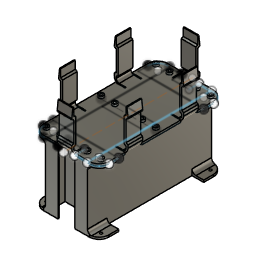
wall_holder (Autodesk Fusion 360 design; units mm, degrees)
Autodesk Fusion 360 part; units mm, degrees
other "Grundnetzelement1"
sketch "Skizze2" plane through (0, 0, 0) normal (0, 0, 1) x (1, 0, 0)
  line L0 (67, -14.1187) -> (67, 146.9687) construction
  line L1 (124.2467, 81.5) -> (-73.8076, 81.5) construction
  line L2 (90.5, 18) -> (43.5, 18)
  line L3 (33.5, 28) -> (33.5, 135)
  line L4 (43.5, 145) -> (90.5, 145)
  line L5 (100.5, 135) -> (100.5, 28)
  line L6 (31.5, 102.5) -> (35.5, 102.5)
  line L7 (35.5, 102.5) -> (35.5, 117.5)
  line L8 (35.5, 117.5) -> (31.5, 117.5)
  line L9 (31.5, 117.5) -> (31.5, 102.5)
  line L10 (59.5, 20) -> (74.5, 20)
  line L11 (74.5, 20) -> (74.5, 16)
  line L12 (74.5, 16) -> (59.5, 16)
  line L13 (59.5, 16) -> (59.5, 20)
  line L14 (35.5, 45.5) -> (31.5, 45.5)
  line L15 (31.5, 45.5) -> (31.5, 60.5)
  line L16 (35.5, 60.5) -> (35.5, 45.5)
  line L17 (31.5, 60.5) -> (35.5, 60.5)
  line L18 (59.5, 147) -> (59.5, 143)
  line L19 (59.5, 143) -> (74.5, 143)
  line L20 (74.5, 143) -> (74.5, 147)
  line L21 (74.5, 147) -> (59.5, 147)
  line L22 (98.5, 102.5) -> (98.5, 117.5)
  line L23 (102.5, 117.5) -> (102.5, 102.5)
  line L24 (98.5, 117.5) -> (102.5, 117.5)
  line L25 (102.5, 102.5) -> (98.5, 102.5)
  line L26 (102.5, 60.5) -> (98.5, 60.5)
  line L27 (98.5, 60.5) -> (98.5, 45.5)
  line L28 (102.5, 45.5) -> (102.5, 60.5)
  line L29 (98.5, 45.5) -> (102.5, 45.5)
  arc A0 (43.5, 145) -> (33.5, 135) centre (43.5, 135) ccw
  arc A1 (100.5, 135) -> (90.5, 145) centre (90.5, 135) ccw
  arc A2 (90.5, 18) -> (100.5, 28) centre (90.5, 28) ccw
  arc A3 (33.5, 28) -> (43.5, 18) centre (43.5, 28) ccw
  circle A4 centre (39, 137.5) radius 2.5
  circle A5 centre (39, 137.5) radius 4.5
  circle A6 centre (53, 137.5) radius 2.5
  circle A7 centre (53, 137.5) radius 4.5
  circle A8 centre (39, 109.5) radius 2.5
  circle A9 centre (39, 109.5) radius 4.5
  circle A10 centre (53, 109.5) radius 2.5
  circle A11 centre (53, 109.5) radius 4.5
  circle A12 centre (39, 81.5) radius 2.5
  circle A13 centre (39, 81.5) radius 4.5
  circle A14 centre (53, 81.5) radius 2.5
  circle A15 centre (53, 81.5) radius 4.5
  circle A16 centre (39, 53.5) radius 2.5
  circle A17 centre (39, 53.5) radius 4.5
  circle A18 centre (53, 53.5) radius 2.5
  circle A19 centre (53, 53.5) radius 4.5
  circle A20 centre (39, 25.5) radius 2.5
  circle A21 centre (39, 25.5) radius 4.5
  circle A22 centre (53, 25.5) radius 2.5
  circle A23 centre (53, 25.5) radius 4.5
  line L30 (41, 137.5) -> (37, 137.5)
  line L31 (37, 137.5) -> (37, 25.5)
  line L32 (37, 25.5) -> (41, 25.5)
  line L33 (41, 25.5) -> (41, 137.5)
  line L34 (39, 137.5) -> (39, 109.5) construction
  line L35 (59.5, 145) -> (58.5, 145)
  line L36 (58.5, 145) -> (58.5, 135)
  line L37 (58.5, 135) -> (59.5, 135)
  line L38 (59.5, 135) -> (59.5, 145)
  line L39 (74.5, 145) -> (75.5, 145)
  line L40 (75.5, 145) -> (75.5, 135)
  line L41 (75.5, 135) -> (74.5, 135)
  line L42 (74.5, 135) -> (74.5, 145)
  line L43 (74.5, 28) -> (74.5, 18)
  line L44 (75.5, 18) -> (75.5, 28)
  line L45 (58.5, 18) -> (58.5, 28)
  line L46 (59.5, 28) -> (59.5, 18)
  line L47 (58.5, 28) -> (59.5, 28)
  line L48 (59.5, 18) -> (58.5, 18)
  line L49 (74.5, 18) -> (75.5, 18)
  line L50 (75.5, 28) -> (74.5, 28)
  line L51 (33.5, 117.5) -> (43.5, 117.5)
  line L52 (43.5, 117.5) -> (43.5, 118.5)
  line L53 (43.5, 118.5) -> (33.5, 118.5)
  line L54 (33.5, 118.5) -> (33.5, 117.5)
  line L55 (33.5, 102.5) -> (43.5, 102.5)
  line L56 (43.5, 102.5) -> (43.5, 101.5)
  line L57 (43.5, 101.5) -> (33.5, 101.5)
  line L58 (33.5, 101.5) -> (33.5, 102.5)
  line L59 (33.5, 61.5) -> (33.5, 60.5)
  line L60 (33.5, 60.5) -> (43.5, 60.5)
  line L61 (43.5, 61.5) -> (33.5, 61.5)
  line L62 (43.5, 60.5) -> (43.5, 61.5)
  line L63 (43.5, 45.5) -> (43.5, 44.5)
  line L64 (33.5, 45.5) -> (43.5, 45.5)
  line L65 (33.5, 44.5) -> (33.5, 45.5)
  line L66 (43.5, 44.5) -> (33.5, 44.5)
  line L67 (90.5, 101.5) -> (100.5, 101.5)
  line L68 (100.5, 102.5) -> (90.5, 102.5)
  line L69 (100.5, 101.5) -> (100.5, 102.5)
  line L70 (90.5, 102.5) -> (90.5, 101.5)
  line L71 (100.5, 118.5) -> (100.5, 117.5)
  line L72 (100.5, 117.5) -> (90.5, 117.5)
  line L73 (90.5, 118.5) -> (100.5, 118.5)
  line L74 (90.5, 117.5) -> (90.5, 118.5)
  line L75 (100.5, 60.5) -> (90.5, 60.5)
  line L76 (90.5, 61.5) -> (100.5, 61.5)
  line L77 (100.5, 61.5) -> (100.5, 60.5)
  line L78 (90.5, 60.5) -> (90.5, 61.5)
  line L79 (90.5, 44.5) -> (100.5, 44.5)
  line L80 (90.5, 45.5) -> (90.5, 44.5)
  line L81 (100.5, 45.5) -> (90.5, 45.5)
  line L82 (100.5, 44.5) -> (100.5, 45.5)
  circle A24 centre (67, 137.5) radius 2.5
  circle A25 centre (67, 137.5) radius 4.5
  circle A26 centre (81, 137.5) radius 2.5
  circle A27 centre (81, 137.5) radius 4.5
  circle A28 centre (95, 137.5) radius 2.5
  circle A29 centre (95, 137.5) radius 4.5
  circle A30 centre (67, 109.5) radius 2.5
  circle A31 centre (67, 109.5) radius 4.5
  circle A32 centre (81, 109.5) radius 2.5
  circle A33 centre (81, 109.5) radius 4.5
  circle A34 centre (95, 109.5) radius 2.5
  circle A35 centre (95, 109.5) radius 4.5
  circle A36 centre (67, 81.5) radius 2.5
  circle A37 centre (67, 81.5) radius 4.5
  circle A38 centre (81, 81.5) radius 2.5
  circle A39 centre (81, 81.5) radius 4.5
  circle A40 centre (95, 81.5) radius 2.5
  circle A41 centre (95, 81.5) radius 4.5
  circle A42 centre (67, 53.5) radius 2.5
  circle A43 centre (67, 53.5) radius 4.5
  circle A44 centre (81, 53.5) radius 2.5
  circle A45 centre (81, 53.5) radius 4.5
  circle A46 centre (95, 53.5) radius 2.5
  circle A47 centre (95, 53.5) radius 4.5
  circle A48 centre (67, 25.5) radius 2.5
  circle A49 centre (67, 25.5) radius 4.5
  circle A50 centre (81, 25.5) radius 2.5
  circle A51 centre (81, 25.5) radius 4.5
  circle A52 centre (95, 25.5) radius 2.5
  circle A53 centre (95, 25.5) radius 4.5
  line L83 (93, 137.5) -> (97, 137.5)
  line L84 (97, 137.5) -> (97, 25.5)
  line L85 (93, 25.5) -> (93, 137.5)
  line L86 (97, 25.5) -> (93, 25.5)
  line L87 (41, 134.5) -> (37, 134.5)
  line L88 (37, 134.5) -> (37, 140.5)
  line L89 (37, 140.5) -> (41, 140.5)
  line L90 (41, 140.5) -> (41, 134.5)
  line L91 (55, 134.5) -> (51, 134.5)
  line L92 (51, 134.5) -> (51, 140.5)
  line L93 (51, 140.5) -> (55, 140.5)
  line L94 (55, 140.5) -> (55, 134.5)
  line L95 (69, 134.5) -> (65, 134.5)
  line L96 (65, 134.5) -> (65, 140.5)
  line L97 (65, 140.5) -> (69, 140.5)
  line L98 (69, 140.5) -> (69, 134.5)
  line L99 (83, 134.5) -> (79, 134.5)
  line L100 (79, 134.5) -> (79, 140.5)
  line L101 (79, 140.5) -> (83, 140.5)
  line L102 (83, 140.5) -> (83, 134.5)
  line L103 (97, 134.5) -> (93, 134.5)
  line L104 (93, 134.5) -> (93, 140.5)
  line L105 (93, 140.5) -> (97, 140.5)
  line L106 (97, 140.5) -> (97, 134.5)
  line L107 (41, 106.5) -> (37, 106.5)
  line L108 (37, 106.5) -> (37, 112.5)
  line L109 (37, 112.5) -> (41, 112.5)
  line L110 (41, 112.5) -> (41, 106.5)
  line L111 (55, 106.5) -> (51, 106.5)
  line L112 (51, 106.5) -> (51, 112.5)
  line L113 (51, 112.5) -> (55, 112.5)
  line L114 (55, 112.5) -> (55, 106.5)
  line L115 (69, 106.5) -> (65, 106.5)
  line L116 (65, 106.5) -> (65, 112.5)
  line L117 (65, 112.5) -> (69, 112.5)
  line L118 (69, 112.5) -> (69, 106.5)
  line L119 (83, 106.5) -> (79, 106.5)
  line L120 (79, 106.5) -> (79, 112.5)
  line L121 (79, 112.5) -> (83, 112.5)
  line L122 (83, 112.5) -> (83, 106.5)
  line L123 (97, 106.5) -> (93, 106.5)
  line L124 (93, 106.5) -> (93, 112.5)
  line L125 (93, 112.5) -> (97, 112.5)
  line L126 (97, 112.5) -> (97, 106.5)
  line L127 (41, 78.5) -> (37, 78.5)
  line L128 (37, 78.5) -> (37, 84.5)
  line L129 (37, 84.5) -> (41, 84.5)
  line L130 (41, 84.5) -> (41, 78.5)
  line L131 (55, 78.5) -> (51, 78.5)
  line L132 (51, 78.5) -> (51, 84.5)
  line L133 (51, 84.5) -> (55, 84.5)
  line L134 (55, 84.5) -> (55, 78.5)
  line L135 (69, 78.5) -> (65, 78.5)
  line L136 (65, 78.5) -> (65, 84.5)
  line L137 (65, 84.5) -> (69, 84.5)
  line L138 (69, 84.5) -> (69, 78.5)
  line L139 (83, 78.5) -> (79, 78.5)
  line L140 (79, 78.5) -> (79, 84.5)
  line L141 (79, 84.5) -> (83, 84.5)
  line L142 (83, 84.5) -> (83, 78.5)
  line L143 (97, 78.5) -> (93, 78.5)
  line L144 (93, 78.5) -> (93, 84.5)
  line L145 (93, 84.5) -> (97, 84.5)
  line L146 (97, 84.5) -> (97, 78.5)
  line L147 (41, 50.5) -> (37, 50.5)
  line L148 (37, 50.5) -> (37, 56.5)
  line L149 (37, 56.5) -> (41, 56.5)
  line L150 (41, 56.5) -> (41, 50.5)
  line L151 (55, 50.5) -> (51, 50.5)
  line L152 (51, 50.5) -> (51, 56.5)
  line L153 (51, 56.5) -> (55, 56.5)
  line L154 (55, 56.5) -> (55, 50.5)
  line L155 (69, 50.5) -> (65, 50.5)
  line L156 (65, 50.5) -> (65, 56.5)
  line L157 (65, 56.5) -> (69, 56.5)
  line L158 (69, 56.5) -> (69, 50.5)
  line L159 (83, 50.5) -> (79, 50.5)
  line L160 (79, 50.5) -> (79, 56.5)
  line L161 (79, 56.5) -> (83, 56.5)
  line L162 (83, 56.5) -> (83, 50.5)
  line L163 (97, 50.5) -> (93, 50.5)
  line L164 (93, 50.5) -> (93, 56.5)
  line L165 (93, 56.5) -> (97, 56.5)
  line L166 (97, 56.5) -> (97, 50.5)
  line L167 (41, 22.5) -> (37, 22.5)
  line L168 (37, 22.5) -> (37, 28.5)
  line L169 (37, 28.5) -> (41, 28.5)
  line L170 (41, 28.5) -> (41, 22.5)
  line L171 (55, 22.5) -> (51, 22.5)
  line L172 (51, 22.5) -> (51, 28.5)
  line L173 (51, 28.5) -> (55, 28.5)
  line L174 (55, 28.5) -> (55, 22.5)
  line L175 (69, 22.5) -> (65, 22.5)
  line L176 (65, 22.5) -> (65, 28.5)
  line L177 (65, 28.5) -> (69, 28.5)
  line L178 (69, 28.5) -> (69, 22.5)
  line L179 (83, 22.5) -> (79, 22.5)
  line L180 (79, 22.5) -> (79, 28.5)
  line L181 (79, 28.5) -> (83, 28.5)
  line L182 (83, 28.5) -> (83, 22.5)
  line L183 (97, 22.5) -> (93, 22.5)
  line L184 (93, 22.5) -> (93, 28.5)
  line L185 (93, 28.5) -> (97, 28.5)
  line L186 (97, 28.5) -> (97, 22.5)
  point P0 (100.5, 18)
  point P1 (33.5, 18)
  point P2 (100.5, 145)
  point P3 (39, 137.5)
  point P4 (53, 137.5)
  point P5 (39, 109.5)
  point P6 (53, 109.5)
  point P7 (39, 81.5)
  point P8 (53, 81.5)
  point P9 (39, 53.5)
  point P10 (53, 53.5)
  point P11 (39, 25.5)
  point P12 (53, 25.5)
  point P13 (35.5, 60.5)
  point P14 (40.3584, 39.5)
  point P15 (35.5, 45.5)
  point P16 (98.5, 102.5)
  point P17 (93.6416, 123.5)
  point P18 (98.5, 117.5)
  point P19 (98.5, 60.5)
  point P20 (98.5, 60.5)
  point P21 (98.5, 45.5)
  point P22 (93.6416, 39.5)
  point P23 (102.5, 45.5)
  point P24 (98.5, 45.5)
  point P25 (93.6416, 36.5)
  point P26 (67, 137.5)
  point P27 (81, 137.5)
  point P28 (95, 137.5)
  point P29 (67, 109.5)
  point P30 (81, 109.5)
  point P31 (95, 109.5)
  point P32 (67, 81.5)
  point P33 (81, 81.5)
  point P34 (95, 81.5)
  point P35 (67, 53.5)
  point P36 (81, 53.5)
  point P37 (95, 53.5)
  point P38 (67, 25.5)
  point P39 (81, 25.5)
  point P40 (95, 25.5)
  dimension "d1" = 67
  dimension "d2" = 127
  dimension "d3" = 67
  dimension "d4" = 81.5
  dimension "d8" = 15
  dimension "d9" = 2
  dimension "d10" = 2
  dimension "d11" = 21
  dimension "d12" = 2
  dimension "d13" = 2
  dimension "d14" = 15
  dimension "d15" = 10
  dimension "d42" = 56
  dimension "d43" = -112
  dimension "d44" = 5
  dimension "d45" = 9
  dimension "d47" = 4
  dimension "d78" = 1
  dimension "d79" = 10
  dimension "d80" = 1
  dimension "d81" = 10
  dimension "d82" = 1
  dimension "d83" = 1
  dimension "d86" = 6
  constraint vertical L0
  constraint horizontal L1
  constraint horizontal L2
  constraint vertical L3
  constraint horizontal L4
  constraint vertical L5
  constraint symmetric L1 L2 L4
  constraint horizontal L6
  constraint vertical L7
  constraint horizontal L8
  constraint vertical L9
  constraint horizontal L10
  constraint vertical L11
  constraint horizontal L12
  constraint vertical L13
  constraint symmetric L1 L6.start L15.end
  constraint symmetric L1 L6.end P13
  constraint symmetric L1 L7.end P15
  constraint symmetric L1 L8.end L14.end
  constraint symmetric L1 L10.start L18.end
  constraint symmetric L1 L10.end L19.end
  constraint symmetric L1 L11.end L20.end
  constraint symmetric L1 L12.end L18.start
  constraint symmetric L0 L6.start L23.end
  constraint symmetric L0 L6.end P16
  constraint symmetric L0 L7.end P18
  constraint symmetric L0 L8.end L23.start
  constraint symmetric L0 P15 P24
  constraint symmetric L0 L14.end P23
  constraint symmetric L0 L15.end L26.start
  constraint symmetric L0 P13 P20
  constraint tangent L4 A0
  constraint tangent L3 A0
  constraint coincident P2 L4
  constraint coincident P2 L5
  constraint tangent L4 A1
  constraint tangent L5 A1
  constraint equal A0 A1
  constraint coincident P0 L2
  constraint coincident P0 L5
  constraint tangent L2 A2
  constraint tangent L5 A2
  constraint equal A0 A2
  constraint coincident P1 L2
  constraint coincident P1 L3
  constraint tangent L2 A3
  constraint tangent L3 A3
  constraint equal A0 A3
  constraint coincident P3 A4.centre
  constraint horizontal L30
  constraint vertical L31
  constraint horizontal L32
  constraint vertical L33
  constraint coincident P5 A8.centre
  constraint horizontal L35
  constraint vertical L36
  constraint horizontal L37
  constraint vertical L38
  constraint coincident L18 L35.start
  constraint coincident L4 L35.start
  constraint horizontal L39
  constraint vertical L40
  constraint horizontal L41
  constraint vertical L42
  constraint coincident L4 L39.start
  constraint coincident L20 L39.start
  constraint collinear L37 L41
  constraint symmetric L1 L35.start L46.end
  constraint symmetric L1 L35.end L45.start
  constraint symmetric L1 L36.end L45.end
  constraint symmetric L1 L37.end L46.start
  constraint symmetric L1 L39.start L43.end
  constraint symmetric L1 L39.end L44.start
  constraint symmetric L1 L40.end L44.end
  constraint symmetric L1 L41.end L43.start
  constraint horizontal L51
  constraint vertical L52
  constraint horizontal L53
  constraint vertical L54
  constraint coincident L3 L51.start
  constraint coincident L8 L51.start
  constraint horizontal L55
  constraint vertical L56
  constraint horizontal L57
  constraint vertical L58
  constraint coincident L3 L55.start
  constraint coincident L6 L55.start
  constraint collinear L52 L56
  constraint symmetric L1 L51.start L64.start
  constraint symmetric L1 L51.end L63.start
  constraint symmetric L1 L52.end L63.end
  constraint symmetric L1 L53.end L65.start
  constraint symmetric L1 L55.start L59.end
  constraint symmetric L1 L55.end L60.end
  constraint symmetric L1 L56.end L61.start
  constraint symmetric L1 L57.end L59.start
  constraint symmetric L0 L51.start L71.end
  constraint symmetric L0 L51.end L72.end
  constraint symmetric L0 L52.end L73.start
  constraint symmetric L0 L53.end L71.start
  constraint symmetric L0 L55.start L68.start
  constraint symmetric L0 L55.end L68.end
  constraint symmetric L0 L56.end L67.start
  constraint symmetric L0 L57.end L67.end
  constraint symmetric L0 L59.end L75.start
  constraint symmetric L0 L59.start L76.end
  constraint symmetric L0 L60.end L75.end
  constraint symmetric L0 L61.start L76.start
  constraint symmetric L0 L65.start L79.end
  constraint symmetric L0 L63.end L79.start
  constraint symmetric L0 L63.start L80.start
  constraint symmetric L0 L64.start L81.start
  constraint symmetric L0 P14 P22
  constraint symmetric L0 A5 A29
  constraint symmetric L1 A5 A21
  constraint symmetric L1 L30 L32
  constraint coincident P3 L30
  constraint symmetric L0 L30.start L83.start
  constraint symmetric L0 L30.end L83.end
  constraint symmetric L0 L31.end L84.end
  constraint symmetric L0 L32.end L85.start
  constraint horizontal L87
  constraint vertical L88
  constraint horizontal L89
  constraint vertical L90
  constraint collinear L31 L88
  constraint collinear L33 L90
  constraint symmetric L30 L87 L89
  measures "d1" distance of P0 P1
  measures "d2" distance of P0 P2
  measures "d3" distance of origin L0
  measures "d4" distance of origin L1
  measures "d8" distance of L6.start L8.end
  measures "d9" distance of L3 L9
  measures "d10" distance of L3 L7
  measures "d11" distance of L1 L6
  measures "d12" distance of L2 L12
  measures "d13" distance of L2 L10
  measures "d14" distance of L11.end L12.end
  measures "d15" radius of A0
  measures "d44" diameter of A4
  measures "d45" diameter of A5
  measures "d47" distance of L31 L33
  measures "d78" distance of L35.start L35.end
  measures "d79" distance of L35.start L37.end
  measures "d80" distance of L39.start L39.end
  measures "d81" distance of L51.start L51.end
  measures "d82" distance of L51.start L53.end
  measures "d83" distance of L55.start L57.end
  measures "d86" distance of L87 L89
extrude "Extrusion1" add sketch "Skizze2" along normal blind -4 and the other way blind 2 contours L2 L3 L4 L5 L10 L19 A0 A1 A2 A3 A5 A9 A13 A17 A21 L31 L33 L36 L37 L38 L40 L41 L42 L43 L44 L45 L46 L47 L50 L51 L52 L53 L55 L56 L57 L60 L61 L62 L63 L64 L66 L67 L68 L70 L72 L73 L74 L75 L76 L78 L79 L80 L81 A29 A35 A41 A47 A53 L84 L85 | L2 L10 L11 L13 L43 L46 | L5 L26 L27 L29 L75 L81 A47 | L79 A53 L84 L85 | L27 L81 A47 L84 | L81 A47 L84 L85 | A53 L84 L85 L185 | A52 A53 L84 L85 L183 L184 L186 | L5 L67 L76 A41 L84 | L27 L75 A47 L84 | L27 A46 A47 L84 L166 | L27 A47 | A47 L84 L85 L163 | A52 L84 L85 L184 L185 L186 | L76 A41 L84 L85 | L75 A47 L84 L85 | A46 A47 L85 L164 | A46 L84 L85 L163 L164 L166 | A52 L84 L85 L86 L184 L186 | A52 L84 L186 | L5 L22 L24 L25 L68 L72 A35 | L67 A41 L84 L85 | A40 A41 L84 L146 | A41 L84 L85 L143 | A47 L84 L85 L165 | A52 L85 L184 | A46 L84 L166 | A46 L84 L85 L164 L166 | A52 L86 L184 L186 | L3 L14 L16 L17 A17 L60 L64 | A21 L31 L33 L66 | L22 L68 A35 L84 | L68 A35 L84 L85 | A41 L84 L85 L145 | A40 A41 L85 L144 | A40 L84 L85 L143 L144 L146 | A46 L84 L85 L164 L165 L166 | A52 L183 L184 L186 | A46 L85 L164 | L16 A17 L31 L64 | A17 L31 L33 L64 | A20 A21 L31 L33 L167 L168 L170 | A21 L31 L33 L169 | L22 L72 A35 L84 | L22 A34 A35 L84 L126 | L22 A35 | A35 L84 L85 L123 | A40 L84 L85 L144 L145 L146 | A40 L84 L146 | A40 L84 L85 L144 L146 | L3 A13 L31 L57 L61 | L16 A17 L31 L60 | L16 A17 | L16 A16 A17 L31 L148 | A17 L31 L33 L147 | A20 L31 L33 L168 L169 L170 | L73 A29 L84 L85 | L72 A35 L84 L85 | A34 A35 L85 L124 | A34 L84 L85 L123 L124 L126 | A40 L85 L144 | A13 L31 L33 L61 | A17 L31 L33 L60 | A16 A17 L33 L150 | A16 L31 L33 L147 L148 L150 | A20 L31 L168 | A20 L31 L32 L33 L168 L170 | A28 A29 L84 L85 L104 L105 L106 | A29 L84 L85 L103 | A35 L84 L85 L125 | A34 L84 L126 | A34 L84 L85 L124 L126 | L3 L6 L7 L8 A9 L51 L55 | A13 L31 L33 L57 | A13 L31 L33 L127 | A12 A13 L31 L128 | A17 L31 L33 L149 | A16 L31 L33 L148 L150 | A16 L31 L148 | A20 L33 L170 | A20 L32 L168 L170 | A20 L167 L168 L170 | A28 L84 L85 L103 L104 L106 | A34 L84 L85 L124 L125 L126 | A34 L85 L124 | L7 A9 L31 L55 | A9 L31 L33 L55 | A13 L31 L33 L129 | A12 A13 L33 L130 | A12 L31 L33 L127 L128 L130 | A16 L31 L33 L148 L149 L150 | A16 L33 L150 | L4 L18 L19 L20 L38 L42 | A28 L84 L106 | A28 L83 L84 L85 L104 L106 | L7 A9 L31 L51 | L7 A9 | L7 A8 A9 L31 L108 | A9 L31 L33 L107 | A12 L31 L33 L128 L129 L130 | A12 L31 L33 L128 L130 | A12 L31 L128 | A28 L85 L104 | A28 L83 L104 L106 | A5 L31 L33 L53 | A9 L31 L33 L51 | A8 A9 L33 L110 | A8 L31 L33 L107 L108 L110 | A12 L33 L130 | A28 L104 L105 L106 | A5 L31 L33 L87 | A4 A5 L31 L33 L88 L89 L90 | A9 L31 L33 L109 | A8 L31 L33 L108 L110 | A8 L31 L108 | A4 L31 L33 L87 L88 L90 | A8 L31 L33 L108 L109 L110 | A8 L33 L110 | A4 L30 L31 L33 L88 L90 | A4 L31 L88 | A4 L33 L90 | A4 L88 L89 L90 | A4 L30 L88 L90 | A6 L94 | A6 L92 L94 | A6 L92 L93 L94 | A6 L91 L92 L94 | A6 L92 | A7 | A10 L114 | A10 L112 L114 | A10 L112 L113 L114 | A10 L111 L112 L114 | A10 L112 | A11 | A14 L134 | A14 L132 L134 | A14 L132 L133 L134 | A14 L131 L132 L134 | A14 L132 | A15 | A18 L154 | A18 L152 L154 | A18 L152 L153 L154 | A18 L151 L152 L154 | A18 L152 | A19 | A22 L174 | A22 L172 L174 | A22 L172 L173 L174 | A22 L171 L172 L174 | A22 L172 | A23 | A24 L98 | A24 L96 L98 | A24 L96 L97 L98 | A24 L95 L96 L98 | A24 L96 | A25 | A26 L102 | A26 L100 L102 | A26 L100 L101 L102 | A26 L99 L100 L102 | A26 L100 | A27 | A30 L118 | A30 L116 L118 | A30 L116 L117 L118 | A30 L115 L116 L118 | A30 L116 | A31 | A32 L122 | A32 L120 L122 | A32 L120 L121 L122 | A32 L119 L120 L122 | A32 L120 | A33 | A36 L138 | A36 L136 L138 | A36 L136 L137 L138 | A36 L135 L136 L138 | A36 L136 | A37 | A38 L142 | A38 L140 L142 | A38 L140 L141 L142 | A38 L139 L140 L142 | A38 L140 | A39 | A42 L158 | A42 L156 L158 | A42 L156 L157 L158 | A42 L155 L156 L158 | A42 L156 | A43 | A44 L162 | A44 L160 L162 | A44 L160 L161 L162 | A44 L159 L160 L162 | A44 L160 | A45 | A48 L178 | A48 L176 L178 | A48 L176 L177 L178 | A48 L175 L176 L178 | A48 L176 | A49 | A50 L182 | A50 L180 L182 | A50 L180 L181 L182 | A50 L179 L180 L182 | A50 L180 | A51 makes body 1
extrude "Extrusion2" add sketch "Skizze2" against normal blind 4 contours L2 L11 L12 L13 | L5 L26 L28 L29 | L5 L23 L24 L25 | L3 L14 L15 L17 | L3 L6 L8 L9 | L4 L18 L20 L21 bodies 1
extrude "Extrusion3" add sketch "Skizze2" along normal blind 38 and the other way blind 0 contours L2 L11 L12 L13 | L5 L26 L28 L29 | L5 L23 L24 L25 | L3 L14 L15 L17 | L3 L6 L8 L9 | L4 L18 L20 L21 bodies 1
extrude "Extrusion4" add sketch "Skizze2" along normal blind 30 and the other way blind -3 contours L2 L10 L11 L13 L43 L46 | L5 L26 L27 L29 L75 L81 A47 | L27 A47 | L5 L22 L24 L25 L68 L72 A35 | L3 L14 L16 L17 A17 L60 L64 | L22 A35 | L16 A17 | L3 L6 L7 L8 A9 L51 L55 | L4 L18 L19 L20 L38 L42 | L7 A9 bodies 1
extrude "Extrusion9" cut sketch "Skizze2" along normal blind 27 and the other way blind -6 contours L2 L11 L12 L13 | L5 L26 L28 L29 | L5 L23 L24 L25 | L3 L14 L15 L17 | L3 L6 L8 L9 | L4 L18 L20 L21 bodies 1
fillet "Abrundung2" radius 6 6 edges at (102.5, 53, -4) (67, 16, -4) (102.5, 110, -4) (31.5, 53, -4) (31.5, 110, -4) (67, 147, -4) on bodies 1
fillet "Abrundung4" radius 3 6 edges at (67, 18, -2) (100.5, 53, -2) (100.5, 110, -2) (67, 145, -2) (33.5, 110, -2) (33.5, 53, -2) on bodies 1
extrude "Extrusion5" add sketch "Skizze2" against normal blind 2 contours A52 L84 L85 L86 L184 L186 | A52 L84 L186 | A52 L85 L184 | A52 L86 L184 L186 | A40 L84 L146 | A40 L84 L85 L144 L146 | A40 L85 L144 | A20 L31 L168 | A20 L31 L32 L33 L168 L170 | A20 L33 L170 | A20 L32 L168 L170 | A28 L84 L106 | A28 L83 L84 L85 L104 L106 | A12 L31 L33 L128 L130 | A12 L31 L128 | A28 L85 L104 | A28 L83 L104 L106 | A12 L33 L130 | A4 L30 L31 L33 L88 L90 | A4 L31 L88 | A4 L33 L90 | A4 L30 L88 L90 | A6 L94 | A6 L92 L94 | A6 L92 | A14 L134 | A14 L132 L134 | A14 L132 | A22 L174 | A22 L172 L174 | A22 L172 | A26 L102 | A26 L100 L102 | A26 L100 | A38 L142 | A38 L140 L142 | A38 L140 | A50 L182 | A50 L180 L182 | A50 L180 bodies 1
hole "Bohrung1" at (95, 81.5, 0) at (95, 25.5, 0) at (39, 137.5, 0) at (81, 137.5, 0) at (53, 137.5, 0) at (81, 25.5, 0) at (53, 25.5, 0) at (81, 81.5, 0) at (53, 81.5, 0) at (39, 25.5, 0) at (39, 81.5, 0) at (95, 137.5, 0) direction (0, 0, -1) diameter 2.529 depth 10 tip angle 118 bodies 1
thread "Gewinde1" "ISO Metric profile 3.0 M3x0.5 6H" major diameter 3.086 minor diameter 2.529 pitch 0.5 angle 60 resizes the face on face at (93.7359, 137.5315, -1.3333) on face at (81.2506, 80.2606, -1.3333) on face at (95.2506, 24.2606, -1.3333) on face at (37.7359, 137.5315, -1.3333) on face at (52.1872, 24.5313, -1.3333) on face at (51.7359, 137.5315, -1.3333) on face at (79.7359, 137.5315, -1.3333) on face at (95.2506, 80.2606, -1.3333) on face at (51.7453, 81.3428, -1.3333) on face at (81.2506, 24.2606, -1.3333) on face at (37.7453, 81.3428, -1.3333) on face at (38.1872, 24.5313, -1.3333) on bodies 1
chamfer "Fase4" distance 1 distance2 2 6 edges at (102.5, 53, 27) (67, 16, 27) (102.5, 110, 27) (31.5, 110, 27) (31.5, 53, 27) (67, 147, 27) measured on face at (102.5, 50.5, 30.6667) measured on face at (69.5, 16, 30.6667) measured on face at (102.5, 112.5, 30.6667) measured on face at (31.5, 112.5, 30.6667) measured on face at (31.5, 50.5, 30.6667) measured on face at (69.5, 147, 30.6667) on bodies 1
chamfer "Fase4" distance 1 distance2 2 6 edges at (102.5, 53, 6) (31.5, 53, 6) (67, 16, 6) (31.5, 110, 6) (102.5, 110, 6) (67, 147, 6) measured on face at (102.5, 50.5, 4.6667) measured on face at (31.5, 50.5, 4.6667) measured on face at (69.5, 16, 4.6667) measured on face at (31.5, 112.5, 4.6667) measured on face at (102.5, 112.5, 4.6667) measured on face at (69.5, 147, 4.6667) on bodies 1
chamfer "Fase4" distance 1 distance2 2 6 edges at (98.5, 53, 3) (35.5, 110, 3) (67, 143, 3) (98.5, 110, 3) (35.5, 53, 3) (67, 20, 3) measured on face at (98.5, 55.5, 12) measured on face at (35.5, 107.5, 12) measured on face at (64.5, 143, 12) measured on face at (98.5, 107.5, 12) measured on face at (35.5, 55.5, 12) measured on face at (64.5, 20, 12) on bodies 1
chamfer "Fase4" distance 2 distance2 1 6 edges at (98.5, 53, 30) (98.5, 110, 30) (67, 20, 30) (67, 143, 30) (35.5, 110, 30) (35.5, 53, 30) measured on face at (99.8333, 50.5, 30) measured on face at (99.8333, 107.5, 30) measured on face at (64.5, 19.3333, 30) measured on face at (64.5, 143.6667, 30) measured on face at (34.1667, 112.5, 30) measured on face at (34.8333, 50.5, 30) on bodies 1
chamfer "Fase6" distance 1 distance2 9 6 edges at (67, 147, 38) (102.5, 110, 38) (102.5, 53, 38) (31.5, 110, 38) (31.5, 53, 38) (67, 16, 38) measured on face at (64.5, 145.6667, 38) measured on face at (101.1667, 112.5, 38) measured on face at (101.1667, 55.5, 38) measured on face at (32.8333, 107.5, 38) measured on face at (32.1667, 55.5, 38) measured on face at (64.5, 17.3333, 38) on bodies 1
sketch "Skizze4" plane through (0, 0, -4) normal (0, 0, -1) x (1, 0, 0)
  circle A0 centre (39, -81.5) radius 1.2645
  circle A1 centre (53, -81.5) radius 1.2645
  circle A2 centre (53, -25.5) radius 1.2645
  circle A3 centre (53, -137.5) radius 1.2645
  circle A4 centre (39, -137.5) radius 1.2645
  circle A5 centre (95, -81.5) radius 1.2645
  circle A6 centre (95, -25.5) radius 1.2645
  circle A7 centre (81, -137.5) radius 1.2645
  circle A8 centre (81, -25.5) radius 1.2645
  circle A9 centre (81, -81.5) radius 1.2645
  circle A10 centre (39, -25.5) radius 1.2645
  circle A11 centre (95, -137.5) radius 1.2645
  line L0 (59.5, -141) -> (74.5, -141)
  line L1 (74.5, -141) -> (74.5, -135)
  line L2 (74.5, -135) -> (75.5, -135)
  line L3 (75.5, -135) -> (75.5, -145)
  line L4 (75.5, -145) -> (90.5, -145)
  arc A12 (90.5, -145) -> (100.5, -135) centre (90.5, -135) ccw
  line L5 (100.5, -135) -> (100.5, -118.5)
  line L6 (100.5, -118.5) -> (90.5, -118.5)
  line L7 (90.5, -118.5) -> (90.5, -117.5)
  line L8 (90.5, -117.5) -> (96.5, -117.5)
  line L9 (96.5, -117.5) -> (96.5, -102.5)
  line L10 (96.5, -102.5) -> (90.5, -102.5)
  line L11 (90.5, -102.5) -> (90.5, -101.5)
  line L12 (90.5, -101.5) -> (100.5, -101.5)
  line L13 (100.5, -101.5) -> (100.5, -61.5)
  line L14 (100.5, -61.5) -> (90.5, -61.5)
  line L15 (90.5, -61.5) -> (90.5, -60.5)
  line L16 (90.5, -60.5) -> (96.5, -60.5)
  line L17 (96.5, -60.5) -> (96.5, -45.5)
  line L18 (96.5, -45.5) -> (90.5, -45.5)
  line L19 (90.5, -45.5) -> (90.5, -44.5)
  line L20 (90.5, -44.5) -> (100.5, -44.5)
  line L21 (100.5, -44.5) -> (100.5, -28)
  arc A13 (100.5, -28) -> (90.5, -18) centre (90.5, -28) ccw
  line L22 (90.5, -18) -> (75.5, -18)
  line L23 (75.5, -18) -> (75.5, -28)
  line L24 (75.5, -28) -> (74.5, -28)
  line L25 (74.5, -28) -> (74.5, -22)
  line L26 (74.5, -22) -> (59.5, -22)
  line L27 (59.5, -22) -> (59.5, -28)
  line L28 (59.5, -28) -> (58.5, -28)
  line L29 (58.5, -28) -> (58.5, -18)
  line L30 (58.5, -18) -> (43.5, -18)
  arc A14 (43.5, -18) -> (33.5, -28) centre (43.5, -28) ccw
  line L31 (33.5, -28) -> (33.5, -44.5)
  line L32 (33.5, -44.5) -> (43.5, -44.5)
  line L33 (43.5, -44.5) -> (43.5, -45.5)
  line L34 (43.5, -45.5) -> (37.5, -45.5)
  line L35 (37.5, -45.5) -> (37.5, -60.5)
  line L36 (37.5, -60.5) -> (43.5, -60.5)
  line L37 (43.5, -60.5) -> (43.5, -61.5)
  line L38 (43.5, -61.5) -> (33.5, -61.5)
  line L39 (33.5, -61.5) -> (33.5, -101.5)
  line L40 (33.5, -101.5) -> (43.5, -101.5)
  line L41 (43.5, -101.5) -> (43.5, -102.5)
  line L42 (43.5, -102.5) -> (37.5, -102.5)
  line L43 (37.5, -102.5) -> (37.5, -117.5)
  line L44 (37.5, -117.5) -> (43.5, -117.5)
  line L45 (43.5, -117.5) -> (43.5, -118.5)
  line L46 (43.5, -118.5) -> (33.5, -118.5)
  line L47 (33.5, -118.5) -> (33.5, -135)
  arc A15 (33.5, -135) -> (43.5, -145) centre (43.5, -135) ccw
  line L48 (43.5, -145) -> (58.5, -145)
  line L49 (58.5, -145) -> (58.5, -135)
  line L50 (58.5, -135) -> (59.5, -135)
  line L51 (59.5, -135) -> (59.5, -141)
  line L52 (58.5, -18) -> (43.5, -18)
  line L53 (58.5, -18) -> (58.5, -28)
  line L54 (75.5, -28) -> (58.5, -28)
  arc A16 (43.5, -18) -> (33.5, -28) centre (43.5, -28) ccw
  line L55 (33.5, -28) -> (33.5, -38)
  line L56 (100.5, -38) -> (33.5, -38)
  line L57 (45.5, -18) -> (45.5, -38)
  line L58 (39, -81.5) -> (95, -81.5) construction
  line L59 (67, -147) -> (67, -15) construction
  line L60 (75.5, -18) -> (75.5, -28)
  line L61 (75.5, -18) -> (90.5, -18)
  arc A17 (100.5, -28) -> (90.5, -18) centre (90.5, -28) ccw
  line L62 (100.5, -28) -> (100.5, -38)
  line L63 (88.5, -18) -> (88.5, -38)
  line L64 (46.5, -19) -> (46.5, -37)
  line L65 (46.5, -37) -> (87.5, -37)
  line L66 (87.5, -37) -> (87.5, -19)
  line L67 (87.5, -19) -> (75.5, -19)
  line L68 (46.5, -19) -> (58.5, -19)
  line L69 (100.5, -125) -> (33.5, -125)
  line L70 (45.5, -145) -> (45.5, -125)
  line L71 (46.5, -144) -> (46.5, -126)
  line L72 (46.5, -126) -> (87.5, -126)
  line L73 (88.5, -145) -> (88.5, -125)
  line L74 (87.5, -126) -> (87.5, -144)
  line L75 (87.5, -144) -> (75.5, -144)
  line L76 (46.5, -144) -> (58.5, -144)
  line L77 (58.5, -145) -> (43.5, -145)
  line L78 (75.5, -145) -> (90.5, -145)
  line L79 (75.5, -135) -> (58.5, -135)
  line L80 (75.5, -145) -> (75.5, -135)
  line L81 (58.5, -145) -> (58.5, -135)
  line L82 (33.5, -135) -> (33.5, -125)
  arc A18 (33.5, -135) -> (43.5, -145) centre (43.5, -135) ccw
  line L83 (100.5, -135) -> (100.5, -125)
  arc A19 (90.5, -145) -> (100.5, -135) centre (90.5, -135) ccw
  line L84 (88.5, -125) -> (88.5, -38)
  line L85 (45.5, -125) -> (45.5, -38)
  line L86 (46.5, -37) -> (46.5, -126)
  line L87 (87.5, -126) -> (87.5, -37)
  line L88 (87.5, -87.5) -> (46.5, -87.5)
  line L89 (46.5, -87.5) -> (46.5, -75.5)
  line L90 (46.5, -75.5) -> (87.5, -75.5)
  line L91 (87.5, -75.5) -> (87.5, -87.5)
  dimension "d143" = 10
  dimension "d144" = 12
  dimension "d146" = 1
  dimension "d147" = 1
  dimension "d148" = 1
  dimension "d149" = 1
  dimension "d150" = 1
  dimension "d159" = 12
  constraint coincident L29.end L30.start
  constraint coincident L30.end A14.start
  constraint coincident L28.end L29.start
  constraint coincident L23.end L24.start
  constraint coincident A14.end L31.start
  constraint coincident L31 L55.end
  constraint parallel L31 L55
  constraint coincident L21 L56.start
  constraint perpendicular L55 L56
  constraint coincident L52 L57.start
  constraint coincident L56 L57.end
  constraint perpendicular L56 L57
  constraint coincident A0.centre L58.start
  constraint coincident A5.centre L58.end
  constraint perpendicular L56 L59
  constraint symmetric L29.end L59 L22.end
  constraint symmetric L30.end L59 A13.end
  constraint symmetric L28.end L59 L23.end
  constraint symmetric A14.end L59 L21.end
  constraint symmetric A16 L59 A17
  constraint symmetric L55.end L59 L56.start
  constraint symmetric L57.start L59 L63.start
  constraint symmetric L57.end L59 L63.end
  constraint perpendicular L64 L65
  constraint perpendicular L65 L66
  constraint coincident L60 L67.end
  constraint perpendicular L60 L67
  constraint coincident L53 L68.end
  constraint perpendicular L53 L68
  constraint symmetric L29.end L58 L48.end
  constraint symmetric L30.end L58 A15.end
  constraint symmetric L28.end L58 L49.end
  constraint symmetric L23.end L58 L2.end
  constraint symmetric A14.end L58 L47.end
  constraint symmetric A16 L58 A18
  constraint symmetric L55.end L58 L69.end
  constraint symmetric L56.start L58 L69.start
  constraint symmetric L57.start L58 L70.start
  constraint symmetric L57.end L58 L70.end
  constraint symmetric L58 L22.end L3.end
  constraint symmetric L58 L23.end L2.end
  constraint symmetric L58 A13.end L4.end
  constraint symmetric L58 L21.end A12.end
  constraint symmetric L58 A17 A19
  constraint symmetric L58 L56.start L69.start
  constraint symmetric L58 L63.start L73.start
  constraint symmetric L58 L63.end L73.end
  constraint symmetric L58 L64.start L71.start
  constraint symmetric L58 L64.end L71.end
  constraint symmetric L58 L65.end L72.end
  constraint symmetric L58 L66.end L74.end
  constraint symmetric L58 L67.end L75.end
  constraint symmetric L58 L68.end L76.end
  constraint horizontal L88
  constraint vertical L89
  constraint horizontal L90
  constraint vertical L91
  constraint coincident L86 L89.end
  constraint coincident L87 L88.start
  constraint symmetric L58 L88 L90
  measures "d143" distance of A14.end L55.end
  measures "d144" distance of L55 L57
  measures "d146" distance of L52 L68
  measures "d147" distance of L61 L67
  measures "d148" distance of L56 L65
  measures "d149" distance of L57 L64
  measures "d150" distance of L63 L66
  measures "d159" distance of L88 L90
extrude "Extrusion14" add sketch "Skizze4" along normal blind 2 separate body contours L2 L3 L49 L50 L71 L72 L74 L75 L76 L79 L80 L81 | L48 L49 L69 L70 L71 L76 L77 L81 L86 | L3 L4 L69 L73 L74 L75 L78 L80 L87 | L47 A15 L48 L69 L70 L77 L82 A18 | L69 L72 L86 L87 | L4 A12 L5 L69 L73 L78 L83 A19 | L29 L30 L52 L53 L56 L57 L64 L68 L86 | L30 A14 L31 L52 A16 L55 L56 L57 | L86 L87 L88 L89 L90 L91 | L21 A13 L22 L56 L61 A17 L62 L63 | L22 L23 L56 L60 L61 L63 L66 L67 L87 | L56 L65 L86 L87 | L23 L24 L28 L29 L53 L54 L60 L64 L65 L66 L67 L68 makes body 2 at (64.1667, 34.6667, -4) makes body 3 at (64.1667, 128.3333, -4) makes body 4 at (71.4559, 85.865, -4)
extrude "Extrusion15" add sketch "Skizze4" along normal blind 65 contours L48 L49 L69 L70 L71 L76 L77 L81 L86 | L3 L4 L69 L73 L74 L75 L78 L80 L87 | L69 L72 L86 L87 | L56 L69 L85 L86 L89 | L56 L69 L84 L87 L91 | L29 L30 L52 L53 L56 L57 L64 L68 L86 | L22 L23 L56 L60 L61 L63 L66 L67 L87 | L56 L65 L86 L87 bodies 2 3 4
extrude "Extrusion16" add sketch "Skizze4" along normal blind 65 and the other way blind -63 contours L48 L49 L69 L70 L71 L76 L77 L81 L86 | L3 L4 L69 L73 L74 L75 L78 L80 L87 | L47 A15 L48 L69 L70 L77 L82 A18 | L69 L72 L86 L87 | L4 A12 L5 L69 L73 L78 L83 A19 | L29 L30 L52 L53 L56 L57 L64 L68 L86 | L30 A14 L31 L52 A16 L55 L56 L57 | L21 A13 L22 L56 L61 A17 L62 L63 | L22 L23 L56 L60 L61 L63 L66 L67 L87 | L56 L65 L86 L87 bodies 2 1
fillet "Abrundung8" radius 4 12 edges at (46.5, 81.5, -6) (87.5, 81.5, -6) (67, 37, -6) (67, 126, -6) (45.5, 135, -6) (45.5, 28, -6) (88.5, 28, -6) (88.5, 135, -6) (88.5, 135, -67) (45.5, 135, -67) (45.5, 28, -67) (88.5, 28, -67) on bodies 2
